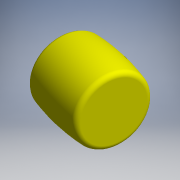
# Autodesk Inventor part: 22205/20 E_r1
Saved by Autodesk Inventor 2017.3 (Build 213256000, 256)
## iProperties
Part Number: 22205/20 E_r1
Material: Generic
Catalog Web Link: www.cadenas.de
Description: BS2_001-Spherical roller bearings
Vendor: SKF
Document SubType Name: Modeling
Designer: partserver
Manufacturer: SKF
Mass: 0.250587 g
Surface Area: 2.08021 cm^2
Volume: 0.250587 cm^3
Density: 1 g/cm^3
Appearance: PSOLRGB-255-255-0
Category: PARTsolutions
Company: SKF
Title: 22205/20 E_r1
Author: Cadenas PARTsolutions
Comments: Spherical roller bearings
PSOL_IDENT_0: {$CADENAS_DATA\23d-libs\skf\bearings_units_and_housings\roller_bearings\spherical_roller_bearings\pa
PSOL_IDENT_1: rts\bs2_001_roller1.prj},171 {VTYP=3D},{NB=22205/20 E_r1},{LINA=22205/20 E_r1},{NN=BS2_001},{DATE=23
PSOL_IDENT_2: .12.2020 11:58:30},{GEOMDATE=24.11.2020 12:16:00},{VERSION=},{LINEID=460970},{WBVAR=},{WBNUMERIC=}
PSOL_IDENT_3: {NB=22205/20 E_r1},{LINA=22205/20 E_r1},{KT=DUMMY},{DESIGNATION=22205/20 E},{VARIANT=CE1W33},{DESIGN
PSOL_IDENT_4: X=Cylindrical bore},{SEAL=No seals},{SALG=NO},{BORE=20.000},{DD=20.000},{DD1=MIN},{D=52.000},{B=18.0
PSOL_IDENT_5: 00},{DD2=31.300},{DD3=MIN},{D1=44.200},{B1=MIN},{B2=MIN},{B4=MIN},{B5=MIN},{BB=3.700},{K=2.000},{R12=
PSOL_IDENT_6: 1.000},{G=},{G1=MIN},{TB=MIN},{ALPHA=12.8333},{R34=MIN},{PITCH=39.459},{DW=7.130},{LW=6.600},{DDAMIN=
PSOL_IDENT_7: 25.600},{DDAMAX=MIN},{DBMIN=MIN},{DAMAX=46.400},{BAMIN=MIN},{RAMAX=1.000},{LOAD1=49.900},{LOAD2=44.0
PSOL_IDENT_8: 00},{LOAD3=4.750},{SPEED1=13000},{SPEED2=17000},{PRA=},{PLA=},{Z=15.000},{II=2.000},{MASS=0.280},{MA
PSOL_IDENT_9: SS2=MIN},{SLEEVE=},{POPULAR=},{BEARING=22205/20 E},{PPATH=parts/bs2_001_asmtpl.prj},{RAMAXX=1},{EE=0
PSOL_IDENT_10: .35},{Y0=1.8},{R12X=1},{Y2=2.9},{ALPHAX=12.83333},{Y1=1.9},{DD1X=},{B1X=},{SLEEVEX=},{ALPHAXX=},{B2X=
PSOL_IDENT_11: },{SUPRESSED=},{BBALG=3.700},{KALG=2.000}
NB: 22205/20 E_r1
NN: BS2_001
NT: Spherical roller bearings
NBSYN: $DESIGNATION._r1
LINA: 22205/20 E_r1
CATALOG: SKF
DESIGNATION: 22205/20 E
VARIANT: CE1W33
DESIGNX: Cylindrical bore
SEAL: No seals
BORE: 20
DD: 20
DD1: 0
D: 52
B: 18
DD2: 31.3
DD3: 0
D1: 44.2
B1: 0
B2: 0
B4: 0
B5: 0
BB: 3.7
K: 2
R12: 1
G1: 0
TB: 0
ALPHA: 12.8333
R34: 0
PITCH: 39.459
DW: 7.13
LW: 6.6
DDAMIN: 25.6
DDAMAX: 0
DBMIN: 0
DAMAX: 46.4
BAMIN: 0
RAMAX: 1
LOAD1: 49.9
LOAD2: 44
LOAD3: 4.75
SPEED1: 13000
SPEED2: 17000
Z: 15
II: 2
MASS: 0.28
MASS2: 0
BEARING: 22205/20 E
PPATH: parts/bs2_001_asmtpl.prj
RAMAXX: 1
EE: 0.35
Y0: 1.8
R12X: 1
Y2: 2.9
ALPHAX: 12.83333
Y1: 1.9
SUPPLIER: SKF
ARTICLENO: 22205/20 E_r1
BOMINFO: 22205/20 E_r1
CREATOR: CADENAS GmbH
Autodesk Inventor part; units mm, degrees
sketch "Sketch_2" plane through (0, 0, 0) normal (0, 0, 1) x (1, 0, 0)
  line L0 (7.7176, 20.4625) -> (1.2824, 18.9965)
  line L1 (1.2824, 18.9965) -> (0.64, 21.8166)
  arc A0 (0.9574, 22.3979) -> (0.64, 21.8166) centre (1.1275, 21.9277) ccw
  arc A1 (6.5373, 23.669) -> (0.9574, 22.3979) centre (8.8822, 0.4928) ccw
  arc A2 (7.0751, 23.2826) -> (6.5373, 23.669) centre (6.5876, 23.1715) ccw
  line L2 (7.0751, 23.2826) -> (7.7176, 20.4625)
  line L3 (7.7176, 20.4625) -> (1.2824, 18.9965)
  constraints: 8 end point, 6 point on circle, 3 centre point
revolve "Revolution1" add sketch "Sketch_2" angle 360 about axis through (7.7176, 20.4625, 0) along (0.9750204, 0.2221152, 0)
ref_plane "NO_GEO_XY" through (0, 0, 0) normal (1, 0, 0) x (0, 0, -1)
ref_plane "NO_GEO_YZ" through (0, 0, 0) normal (0, 0, -1) x (0, 1, 0)
ref_plane "NO_GEO_ZX" through (0, 0, 0) normal (0, 1, 0) x (1, 0, 0)
ref_plane "roller1_XY" through (0, 19.7295, 0) normal (1, 0, 0) x (0, 0, -1)
ref_plane "roller1_YZ" through (0, 19.7295, 0) normal (0, 0, -1) x (0, 1, 0)
ref_plane "roller1_ZX" through (0, 19.7295, 0) normal (0, 1, 0) x (1, 0, 0)
body "Solid1"
